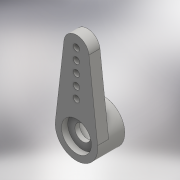
# Autodesk Inventor part: Small Continuous Servo Horn
Saved by Autodesk Inventor 2016 SP2 (Build 200236200, 236)
## iProperties
Created: 2017-09-10
Part Number: Small Continuous Servo Horn
Material: Generic
Document SubType Name: Modeling
Designer: Jared
Density: 1 g/cm^3
Appearance: Default
Author: Jared
Autodesk Inventor part; units mm, degrees
ref_plane "YZ Plane" through (0, 0, 0) normal (1, 0, 0) x (0, 1, 0)
ref_plane "XZ Plane" through (0, 0, 0) normal (0, 1, 0) x (-1, 0, 0)
ref_plane "XY Plane" through (0, 0, 0) normal (0, 0, 1) x (1, 0, 0)
sketch "Sketch1" plane through (0, 0, 0) normal (0, 1, 0) x (-1, 0, 0)
  circle A0 centre (0, 0) radius 3.375
  line L0 (0, -3.375) -> (0, 13.925)
  circle A1 centre (0, 11.925) radius 2
  line L1 (1.9867, 12.1556) -> (3.3525, 0.3892)
  line L2 (-1.9867, 12.1556) -> (-3.3525, 0.3892)
  dimension "d0" = 6.75
  dimension "d1" = 17.3
  dimension "d2" = 4
  constraints: 6 end point, 6 point on circle, 4 tangent, 2 centre point, 1 coincident, 1 point on line, 1 vertical
  measures "d0" diameter of A0
  measures "d1" distance of L0.start L0.end
  measures "d2" diameter of A1
extrude "Extrusion1" add sketch "Sketch1" along normal blind 1.75
sketch "Sketch2" plane through (0, 1.75, 0) normal (0, 1, 0) x (1, 0, 0)
  arc A0 (3.3525, -0.3892) -> (-3.3525, -0.3892) centre (0, 0) ccw projected
  line L0 (-3.3525, -0.3892) -> (-1.9867, -12.1556) projected
  arc A1 (-3.3525, -0.3892) -> (3.3525, -0.3892) centre (0, 0) ccw
  circle A2 centre (0, 0) radius 2.875
  dimension "d5" = 5.75
  constraints: 2 centre point, 2 coincident, 2 point on circle
  measures "d5" diameter of A2
extrude "Extrusion2" add sketch "Sketch2" along normal blind 2.55
sketch "Sketch3" plane through (0, 0, 0) normal (0, -1, 0) x (1, 0, 0)
  arc A0 (-3.3525, 0.3892) -> (3.3525, 0.3892) centre (0, 0) ccw projected
  circle A1 centre (0, 0) radius 2.375
  dimension "d8" = 4.75
  constraints: 1 centre point, 1 coincident
  measures "d8" diameter of A1
extrude "Extrusion3" cut sketch "Sketch3" against normal blind 1
sketch "Sketch4" plane through (0, 1, 0) normal (0, -1, 0) x (1, 0, 0)
  circle A0 centre (0, 0) radius 1.25
  dimension "d11" = 2.5
  constraints: 1 centre point, 1 coincident
  measures "d11" diameter of A0
extrude "Extrusion4" cut sketch "Sketch4" against normal up to next
sketch "Sketch5" plane through (0, 1.75, 0) normal (0, 1, 0) x (1, 0, 0)
  arc A0 (-1.9867, -12.1556) -> (1.9867, -12.1556) centre (0, -11.925) ccw projected
  arc A1 (-3.3525, -0.3892) -> (3.3525, -0.3892) centre (0, 0) ccw projected
  line L0 (0, -3.375) -> (0, -5.1333)
  line L1 (0, -5.1333) -> (0, -6.8917)
  line L2 (0, -6.8917) -> (0, -8.65)
  line L3 (0, -8.65) -> (0, -10.4083)
  line L4 (0, -10.4083) -> (0, -12.1667)
  line L5 (0, -12.1667) -> (0, -13.925)
  constraints: 12 end point, 5 coincident, 5 collinear, 4 point on line, 2 point on circle, 1 vertical
hole "Hole1" at (0, 1.75, 5.1333) at (0, 1.75, 6.8917) at (0, 1.75, 8.65) at (0, 1.75, 10.4083) at (0, 1.75, 12.1667) direction (0, -1, 0) diameter 1 end through all
body "Solid1"
